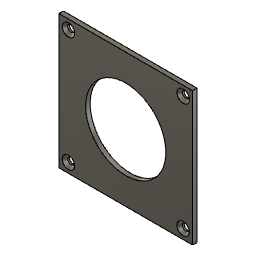
HQ Camera Front v4 (Autodesk Fusion 360 design; units mm, degrees)
Autodesk Fusion 360 part; units mm, degrees
sketch "Sketch1" plane through (0, 0, 0) normal (0, 0, 1) x (1, 0, 0)
  line L0 (-30, 30) -> (30, 30)
  line L1 (30, 30) -> (30, -30)
  line L2 (30, -30) -> (-30, -30)
  line L3 (-30, -30) -> (-30, 30)
  line L4 (-30, 30) -> (30, -30) construction
  line L5 (30, 30) -> (-30, -30) construction
  circle A0 centre (-25.75, 25.75) radius 1.55
  circle A1 centre (25.75, 25.75) radius 1.55
  circle A2 centre (25.76, -25.76) radius 1.55
  circle A3 centre (-25.75, -25.75) radius 1.55
  circle A4 centre (0, 0) radius 18
  dimension "d1" = 60
  dimension "d2" = 60
  dimension "d3" = 3.1
  dimension "d4" = 3.1
  dimension "d5" = 3.1
  dimension "d6" = 3.1
  dimension "d7" = 4.24
  dimension "d8" = 4.25
  dimension "d9" = 4.25
  dimension "d10" = 4.25
  dimension "d11" = 36
  constraint horizontal L0
  constraint perpendicular L0 L1
  constraint parallel L0 L2
  constraint parallel L1 L3
  constraint coincident L4 A4.centre
  constraint coincident L5 A4.centre
  constraint coincident A4.centre origin
  constraint coincident L4 A0.centre
  constraint coincident L5 A1.centre
  constraint coincident L4 A2.centre
  constraint coincident L5 A3.centre
  measures "d1" distance of L1.end L2.end
  measures "d2" distance of L0.end L1.end
  measures "d3" diameter of A0
  measures "d4" diameter of A1
  measures "d5" diameter of A2
  measures "d6" diameter of A3
  measures "d7" distance of L1 A2.centre
  measures "d8" distance of L3 A3.centre
  measures "d9" distance of L3 A0.centre
  measures "d10" distance of L1 A1.centre
  measures "d11" diameter of A4
extrude "Extrude1" add sketch "Sketch1" along normal blind 2
chamfer "Chamfer1" distance 1.25 angle 45 4 edges at (-27.1951, 26.3105, 2) (24.3049, 26.3105, 2) (24.3149, -25.1995, 2) (-27.1951, -25.1895, 2)
